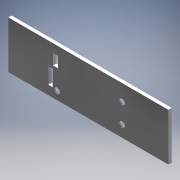
# Autodesk Inventor part: Tyl
Saved by Autodesk Inventor 2019 (Build 230136000, 136)
## iProperties
Created: 2022-02-03
Part Number: Tyl
Material: Aluminium 6061
Document SubType Name: Modeling
Designer: Michał
Density: 2.7 g/cm^3
Appearance: Aluminium — płaski
Mass: 15.0029 g
Surface Area: 61.813 cm^2
Volume: 5.55662 cm^3
Author: Michał
Autodesk Inventor part; units mm, degrees
ref_plane "YZ Plane" through (0, 0, 0) normal (1, 0, 0) x (0, 1, 0)
ref_plane "XZ Plane" through (0, 0, 0) normal (0, 1, 0) x (-1, 0, 0)
ref_plane "XY Plane" through (0, 0, 0) normal (0, 0, 1) x (1, 0, 0)
sketch "Szkic1" plane through (0, 0, 0) normal (1, 0, 0) x (0, 1, 0)
  line L0 (0, 0) -> (0, -2)
  line L1 (0, -2) -> (29, -2)
  line L2 (29, -2) -> (29, 0)
  line L3 (29, 0) -> (0, 0)
  dimension "d0" = 29
  dimension "d1" = 2
  constraints: 8 end point, 3 perpendicular, 1 vertical
  measures "d0" distance between parallel lines of L0 L2
  measures "d1" distance between parallel lines of L3 L1
extrude "Wyciągnięcie proste1" add sketch "Szkic1" along normal blind 98
sketch "Szkic2" plane through (0, 0, -2) normal (0, 0, -1) x (-1, 0, 0)
  line L0 (0, 0) -> (-98, 0) construction
  line L1 (-49, 0) -> (-49, 29) construction
  line L2 (0, 29) -> (-98, 29) construction
  point P0 (-69.65, 19)
  point P1 (-69.65, 7)
  point P2 (-29.85, 5)
  dimension "d4" = 7
  dimension "d5" = 20.65
  dimension "d6" = 19
  dimension "d15" = 19.15
  dimension "d16" = 5
  constraints: 2 end point, 2 midpoint, 1 vertical alignment
  measures "d4" distance from line of L0 point (-69.65, 7)
  measures "d5" distance from line of L1 point (-69.65, 7)
  measures "d6" distance from line of L0 point (-69.65, 19)
  measures "d15" distance from line of L1 point (-29.85, 5)
  measures "d16" distance from line of L0 point (-29.85, 5)
hole "Otwór1" at (69.65, 19, -2) at (69.65, 7, -2) at (29.85, 5, -2) direction (0, 0, 1) diameter 3.4 depth 5.5 tip angle 118 countersink diameter 6.9 countersink angle 84.225 clearance for "Śruba ze łbem stożkowym ISO 2009/7046" size "M3" standard "ISO"
sketch "Szkic3" plane through (0, 0, -2) normal (0, 0, -1) x (-1, 0, 0)
  line L0 (-32.35, 2) -> (-32.35, 27) projected
  line L1 (-27.15, 5.55) -> (-24.45, 5.55)
  line L2 (-24.45, 5.55) -> (-24.45, 15.55)
  line L3 (-24.45, 15.55) -> (-27.15, 15.55)
  line L4 (-27.15, 15.55) -> (-27.15, 5.55)
  line L5 (-30.35, 23.9) -> (-27.35, 23.9)
  line L6 (-27.35, 23.9) -> (-27.35, 17.2)
  line L7 (-27.35, 17.2) -> (-30.35, 17.2)
  line L8 (-30.35, 17.2) -> (-30.35, 23.9)
  point P0 (0, 0)
  dimension "d17" = 5.2
  dimension "d18" = 3.55
  dimension "d19" = 2.7
  dimension "d20" = 10
  dimension "d21" = 2
  dimension "d22" = 15.2
  dimension "d23" = 6.7
  dimension "d24" = 3
  constraints: 16 end point, 4 parallel, 2 horizontal, 2 perpendicular
  measures "d17" distance between parallel lines of L0 L4
  measures "d18" distance from line of L0.start L1
  measures "d19" distance between parallel lines of L2 L4
  measures "d20" distance of L1.end L2.end
  measures "d21" distance between parallel lines of L0 L8
  measures "d22" distance from line of L0.start L7
  measures "d23" distance of L5.end L6.end
  measures "d24" distance of L5.start L5.end
extrude "Wyciągnięcie proste2" cut sketch "Szkic3" against normal up to next
